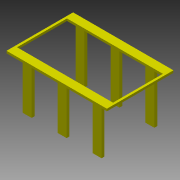
# Autodesk Inventor part: C-0301_pins
Saved by Autodesk Inventor 2014 SP2 (Build 180246200, 246)
## iProperties
Created: 2019-03-13
Part Number: C-0301_pins
Material: Generic
Catalog Web Link: www.cadenas.de
Description: CLT Pins-Pins
Vendor: SAMTEC
Document SubType Name: Modeling
Designer: psadmin
Manufacturer: SAMTEC
Mass: 0.00219327 g
Surface Area: 0.395134 cm^2
Volume: 0.00219327 cm^3
Density: 1 g/cm^3
Appearance: PSOLRGB-255-255-0
Category: PARTsolutions
Company: SAMTEC
Title: C-0301_pins
Author: Cadenas PARTsolutions
Comments: Pins
PSOL_IDENT_0: {$CADENAS_DATA\23d-libs\samtec\modelling\clt\parts\clt_pins.prj},176 {VTYP=3D},{NB=C-0301_pins},{LIN
PSOL_IDENT_1: A=C-0301_pins},{NN=CLT Pins},{DATE=01.08.2018 08:15:54},{GEOMDATE=13.11.2014 08:26:00},{VERSION=},{L
PSOL_IDENT_2: INEID=10},{WBVAR=POS,LS,BEOPT},{WBNUMERIC=}  {NB=C-0301_pins},{LINA=C-0301_pins},{KT=DUMMY},{PN=C-03
PSOL_IDENT_3: 01},{SERIES=CLT},{POSALG=  '02' , '-02' , '03' , '-03' , '04' , '-04' , '05' , '-05' , '06' , '-06'
PSOL_IDENT_4: , '07' , '-07' , '08' , '-08' , '09' , '-09' , '10' , '-10' , '11' , '-11' , '12' , '-12' , '13' , '
PSOL_IDENT_5: -13' , '14' , '-14' , '15' , '-15' , '16' , '-16' , '17' , '-17' , '18' , '-18' , '19' , '-19' , '20'
PSOL_IDENT_6: , '-20' , '21' , '-21' , '22' , '-22' , '23' , '-23' , '24' , '-24' , '25' , '-25' , '26' , '-26' ,
PSOL_IDENT_7: '27' , '-27' , '28' , '-28' , '29' , '-29' , '30' , '-30' , '31' , '-31' , '32' , '-32' , '33' , '-
PSOL_IDENT_8: 33' , '34' , '-34' , '35' , '-35' , '36' , '-36' , '37' , '-37' , '38' , '-38' , '39' , '-39' , '40'
PSOL_IDENT_9: , '-40' , '41' , '-41' , '42' , '-42' , '43' , '-43' , '44' , '-44' , '45' , '-45' , '46' , '-46' ,
PSOL_IDENT_10: '47' , '-47' , '48' , '-48' , '49' , '-49' , '50' , '-50'  },{POS=03},{LS=01},{ROPT=-D},{BEOPT=},{A=
PSOL_IDENT_11: 0.085},{B=0.180},{PINS=3},{H2=0.030},{W=0.120},{PINH=0.131},{PINL=0.085},{PINW=0.020}
NN: CLT Pins
NT: Pins
NB: C-0301_pins
NBSYN: $PN._pins
LINA: C-0301_pins
PN: C-0301
SERIES: CLT
POS: -03
LS: -01
ROPT: -D
BEOPT: Not Selected
A: 0.085
B: 0.18
H2: 0.03
W: 0.12
PINH: 0.131
PINL: 0.085
PINW: 0.02
SUPPLIER: SAMTEC
ARTICLENO: C-0301_pins
BOMINFO: C-0301_pins
CREATOR: CADENAS GmbH
Autodesk Inventor part; units mm, degrees
sketch "Sketch_3" plane through (0, 0.762, 0) normal (0, 1, 0) x (1, 0, 0)
  line L0 (-2.873, 1.905) -> (-2.873, -1.905)
  line L1 (-2.873, -1.905) -> (2.873, -1.905)
  line L2 (2.873, -1.905) -> (2.873, 1.905)
  line L3 (2.873, 1.905) -> (-2.873, 1.905)
  constraints: 8 end point
extrude "Extrusion1" add sketch "Sketch_3" against normal blind 2.921
sketch "Sketch_4" plane through (0, 0.635, 0) normal (0, 1, 0) x (1, 0, 0)
  line L0 (-3, 2.54) -> (-3, -2.54)
  line L1 (-3, -2.54) -> (3, -2.54)
  line L2 (3, -2.54) -> (3, 2.54)
  line L3 (3, 2.54) -> (-3, 2.54)
  line L4 (1.746, -1.4287) -> (1.746, -1.5938)
  line L5 (1.746, -1.5938) -> (2.254, -1.5938)
  line L6 (2.254, -1.5938) -> (2.254, -1.4287)
  line L7 (2.254, -1.4287) -> (1.746, -1.4287)
  line L8 (1.746, 1.5938) -> (1.746, 1.4287)
  line L9 (1.746, 1.4287) -> (2.254, 1.4287)
  line L10 (2.254, 1.4287) -> (2.254, 1.5938)
  line L11 (2.254, 1.5938) -> (1.746, 1.5938)
  line L12 (-0.254, -1.4287) -> (-0.254, -1.5938)
  line L13 (-0.254, -1.5938) -> (0.254, -1.5938)
  line L14 (0.254, -1.5938) -> (0.254, -1.4287)
  line L15 (0.254, -1.4287) -> (-0.254, -1.4287)
  line L16 (-0.254, 1.5938) -> (-0.254, 1.4287)
  line L17 (-0.254, 1.4287) -> (0.254, 1.4287)
  line L18 (0.254, 1.4287) -> (0.254, 1.5938)
  line L19 (0.254, 1.5938) -> (-0.254, 1.5938)
  line L20 (-2.254, -1.4287) -> (-2.254, -1.5938)
  line L21 (-2.254, -1.5938) -> (-1.746, -1.5938)
  line L22 (-1.746, -1.5938) -> (-1.746, -1.4287)
  line L23 (-1.746, -1.4287) -> (-2.254, -1.4287)
  line L24 (-2.254, 1.5938) -> (-2.254, 1.4287)
  line L25 (-2.254, 1.4287) -> (-1.746, 1.4287)
  line L26 (-1.746, 1.4287) -> (-1.746, 1.5938)
  line L27 (-1.746, 1.5938) -> (-2.254, 1.5938)
  constraints: 56 end point
extrude "Extrusion2" cut sketch "Sketch_4" against normal blind 2.921
sketch "Sketch_5" plane through (0, 0, 0) normal (0, 1, 0) x (-1, 0, 0)
  line L0 (2.746, -1.4287) -> (2.746, 1.4287)
  line L1 (2.746, 1.4287) -> (-2.746, 1.4287)
  line L2 (-2.746, 1.4287) -> (-2.746, -1.4287)
  line L3 (-2.746, -1.4287) -> (2.746, -1.4287)
  constraints: 8 end point
extrude "Extrusion3" cut sketch "Sketch_5" along normal blind 2.159
ref_plane "pins_XY" through (0, 0, 0) normal (0, 1, 0) x (1, 0, 0)
ref_plane "pins_YZ" through (0, 0, 0) normal (1, 0, 0) x (0, 0, -1)
ref_plane "pins_ZX" through (0, 0, 0) normal (0, 0, -1) x (0, 1, 0)
body "Solid1"
